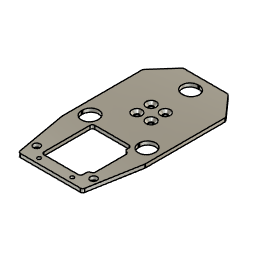
DASHBOARD_PLATE (Autodesk Fusion 360 design; units mm, degrees)
Autodesk Fusion 360 part; units mm, degrees
note: some values were not read from the file. Set by a fixed rule: which sketch regions a step uses.
sketch "Esquisse1" plane through (0, 0, 0) normal (0, 0, 1) x (1, 0, 0)
  circle A0 centre (11, 9.5204) radius 2.85
  circle A1 centre (59, 9.5204) radius 2.85
  line L0 (20.5, 49) -> (49.5, 49)
  line L1 (49.5, 6) -> (20.5, 6)
  line L2 (55, 41) -> (55, 15)
  line L3 (18.5, 47) -> (18.5, 48)
  line L4 (51.5, 47) -> (51.5, 45)
  line L5 (53.5, 43) -> (53, 43)
  line L6 (53, 13) -> (53.5, 13)
  line L7 (51.5, 11) -> (51.5, 8)
  line L8 (18.5, 8) -> (18.5, 9)
  arc A2 (18.5, 8) -> (20.5, 6) centre (20.5, 8) ccw
  arc A3 (49.5, 6) -> (51.5, 8) centre (49.5, 8) ccw
  arc A4 (53.5, 13) -> (51.5, 11) centre (53.5, 11) ccw
  arc A5 (53, 13) -> (55, 15) centre (53, 15) ccw
  arc A6 (55, 41) -> (53, 43) centre (53, 41) ccw
  arc A7 (51.5, 45) -> (53.5, 43) centre (53.5, 45) ccw
  arc A8 (51.5, 47) -> (49.5, 49) centre (49.5, 47) ccw
  arc A9 (20.5, 49) -> (18.5, 47) centre (20.5, 47) ccw
  line L9 (24, 139.2043) -> (24, -40.7957) construction
  line L10 (46, 139.2043) -> (46, -40.7957) construction
  circle A10 centre (29, 88) radius 2
  circle A11 centre (41, 88) radius 2
  circle A12 centre (29, 76) radius 2
  circle A13 centre (41, 76) radius 2
  line L11 (0, 0) -> (0, -3)
  circle A14 centre (49, 1.5) radius 1.5
  circle A15 centre (21, 1.5) radius 1.5
  line L12 (69.9691, 41.8263) -> (62.2933, -1.3501)
  line L13 (0.0309, 41.8263) -> (7.7067, -1.3501)
  line L14 (54.5967, 127.3287) -> (69.4948, 110.5683)
  line L15 (15.4033, 127.3287) -> (0.5052, 110.5683)
  line L16 (16.8981, 128) -> (53.1019, 128)
  line L17 (70, 109.2396) -> (70, 42.1764)
  line L18 (0, 109.2396) -> (0, 42.1764)
  line L19 (9.6758, -3) -> (60.3242, -3)
  arc A16 (0.5052, 110.5683) -> (0, 109.2396) centre (2, 109.2396) ccw
  arc A17 (16.8981, 128) -> (15.4033, 127.3287) centre (16.8981, 126) ccw
  arc A18 (54.5967, 127.3287) -> (53.1019, 128) centre (53.1019, 126) ccw
  arc A19 (70, 109.2396) -> (69.4948, 110.5683) centre (68, 109.2396) ccw
  arc A20 (69.9691, 41.8263) -> (70, 42.1764) centre (68, 42.1764) ccw
  arc A21 (0, 42.1764) -> (0.0309, 41.8263) centre (2, 42.1764) ccw
  arc A22 (60.3242, -3) -> (62.2933, -1.3501) centre (60.3242, -1) ccw
  arc A23 (7.7067, -1.3501) -> (9.6758, -3) centre (9.6758, -1) ccw
  line L20 (34.5, 108.45) -> (35.5, 108.45)
  arc A24 (35.5, 108.45) -> (35.5, 122.05) centre (35.5, 115.25) ccw
  line L21 (35.5, 122.05) -> (34.5, 122.05)
  arc A25 (34.5, 122.05) -> (34.5, 108.45) centre (34.5, 115.25) ccw
  line L22 (34.5, 115.25) -> (35.5, 115.25) construction
  line L23 (65.8, 54.0204) -> (65.8, 55.0204)
  arc A26 (65.8, 55.0204) -> (52.2, 55.0204) centre (59, 55.0204) ccw
  line L24 (52.2, 55.0204) -> (52.2, 54.0204)
  arc A27 (52.2, 54.0204) -> (65.8, 54.0204) centre (59, 54.0204) ccw
  line L25 (59, 54.0204) -> (59, 55.0204) construction
  line L26 (17.8, 54.0204) -> (17.8, 55.0204)
  arc A28 (17.8, 55.0204) -> (4.2, 55.0204) centre (11, 55.0204) ccw
  line L27 (4.2, 55.0204) -> (4.2, 54.0204)
  arc A29 (4.2, 54.0204) -> (17.8, 54.0204) centre (11, 54.0204) ccw
  line L28 (11, 54.0204) -> (11, 55.0204) construction
  line L29 (18.5, 48) -> (18.5, 9)
  point P0 (18.5, 49)
  point P1 (51.5, 49)
  point P2 (18.5, 6)
  point P3 (15, 46)
  point P4 (55, 13)
  point P5 (15, 11)
  point P6 (62, -3)
  point P7 (8, -3)
  point P8 (0, 42)
  point P9 (35, 115.25)
  point P10 (59, 54.5204)
  point P11 (11, 54.5204)
  dimension "d20" = 48
  dimension "d22" = 65.3
  dimension "d23" = 65.3
  dimension "d26" = 5.7
  dimension "d27" = 45
  dimension "d28" = 5.7
  dimension "d29" = 33
  dimension "d37" = 2
  dimension "d38" = 2
  dimension "d40" = 11
  dimension "d41" = 22
  dimension "d42" = 180
  dimension "d43" = 180
  dimension "d56" = 3
  dimension "d63" = 3
  dimension "d64" = 3
  dimension "d66" = 3
  dimension "d68" = 3
  dimension "d71" = 8
  dimension "d72" = 45
  dimension "d77" = 2
  dimension "d78" = 13.6
  dimension "d79" = 1
  dimension "d80" = 13.6
  dimension "d81" = 13.6
  dimension "d82" = 1
  dimension "d83" = 1
  dimension "d84" = 26
  dimension "d86" = 34
  dimension "d92" = 40
  constraint horizontal L0
  constraint horizontal L1
  constraint vertical L2
  constraint perpendicular L0 L3
  constraint perpendicular L0 L4
  constraint perpendicular L2 L5
  constraint perpendicular L2 L6
  constraint perpendicular L1 L7
  constraint perpendicular L1 L8
  constraint coincident P2 L1
  constraint coincident P2 L8
  constraint tangent L1 A2
  constraint tangent L8 A2
  constraint tangent L1 A3
  constraint tangent L7 A3
  constraint tangent L6 A4
  constraint tangent L7 A4
  constraint equal A3 A4
  constraint coincident P4 L2
  constraint coincident P4 L6
  constraint tangent L2 A5
  constraint tangent L6 A5
  constraint equal A3 A5
  constraint tangent L2 A6
  constraint tangent L5 A6
  constraint equal A3 A6
  constraint tangent L4 A7
  constraint tangent L5 A7
  constraint equal A3 A7
  constraint coincident P1 L0
  constraint coincident P1 L4
  constraint tangent L0 A8
  constraint tangent L4 A8
  constraint equal A3 A8
  constraint coincident P0 L0
  constraint coincident P0 L3
  constraint tangent L0 A9
  constraint tangent L3 A9
  constraint equal A3 A9
  constraint coincident L11.start origin
  constraint horizontal L16
  constraint perpendicular L16 L17
  constraint tangent L15 A16
  constraint tangent L18 A16
  constraint tangent L15 A17
  constraint tangent L16 A17
  constraint equal A16 A17
  constraint tangent L14 A18
  constraint tangent L16 A18
  constraint equal A16 A18
  constraint tangent L14 A19
  constraint tangent L17 A19
  constraint equal A16 A19
  constraint tangent L12 A20
  constraint tangent L17 A20
  constraint equal A16 A20
  constraint coincident P8 L13
  constraint coincident P8 L18
  constraint tangent L13 A21
  constraint tangent L18 A21
  constraint equal A16 A21
  constraint coincident P6 L12
  constraint coincident P6 L19
  constraint tangent L12 A22
  constraint tangent L19 A22
  constraint equal A16 A22
  constraint coincident P7 L13
  constraint coincident P7 L19
  constraint tangent L13 A23
  constraint tangent L19 A23
  constraint equal A16 A23
  constraint tangent L20 A24
  constraint tangent A24 L21
  constraint parallel L20 L21
  constraint tangent L21 A25
  constraint tangent L20 A25
  constraint horizontal L22
  constraint midpoint L22 P9
  constraint tangent L23 A26
  constraint tangent A26 L24
  constraint parallel L23 L24
  constraint tangent L24 A27
  constraint tangent L23 A27
  constraint parallel L10 L25
  constraint midpoint L25 P10
  constraint tangent L26 A28
  constraint tangent A28 L27
  constraint parallel L26 L27
  constraint tangent L27 A29
  constraint tangent L26 A29
  constraint vertical L28
  constraint midpoint L28 P11
  constraint parallel L8 L29
  measures "d20" distance of P10 P11
  measures "d22" distance of P9 P10
  measures "d23" distance of P9 P11
  measures "d26" diameter of A0
  measures "d27" distance of A1.centre P10
  measures "d28" diameter of A1
  measures "d29" distance of P0 P1
  measures "d37" radius of A2
  measures "d38" radius of A3
  measures "d40" horizontal distance of L10.start P9
  measures "d41" distance of L10.start L9.start
  measures "d42" distance of L9.start L9.end
  measures "d43" distance of L10.start L10.end
  measures "d56" distance of L11.start L11.end
  measures "d63" diameter of A14
  measures "d64" distance of L10 A14.centre
  measures "d66" diameter of A15
  measures "d68" distance of L9 A15.centre
  measures "d71" distance of L11.end P7
  measures "d72" distance of L11.end P8
  measures "d77" radius of A16
  measures "d78" distance of L20 L21
  measures "d79" distance of A25.centre A24.centre
  measures "d80" diameter of A26
  measures "d81" diameter of A28
  measures "d82" distance of A27.centre A26.centre
  measures "d83" distance of A29.centre A28.centre
  measures "d84" distance of A5.centre A6.centre
  measures "d86" distance of L0 A5.centre
  measures "d92" distance of A11.centre L16
extrude "Extrusion1" add sketch "Esquisse1" along normal blind 3
chamfer "Chanfrein1" distance 2.2 angle 45 4 edges at (27.1353, 76.7232, 3) (27.1353, 88.7232, 3) (39.1353, 76.7232, 3) (39.1353, 88.7232, 3)
